Autodesk Fusion 360 part; units mm, degrees
(part 2 of 2)
sketch "Sketch11" plane through (0, 0, 0) normal (0, -1, 0) x (1, 0, 0)
  arc A0 (-10.5, 6.5391) -> (-5.9173, 0.7089) centre (-4.5, 6.5391) ccw
  arc A1 (-5.9173, 0.7089) -> (5.9173, 0.7089) centre (0, 25.0499) ccw
  arc A2 (5.9173, 0.7089) -> (10.5, 6.5391) centre (4.5, 6.5391) ccw
  line L0 (10.5, 6.5391) -> (10.5, 12.3068)
  line L1 (10.5, 12.3068) -> (-10.5, 12.3068)
  line L2 (-10.5, 12.3068) -> (-10.5, 6.5391)
  line L3 (10.5, 12.3068) -> (11.8, 12.3068)
  line L4 (13, 11.1068) -> (13, 10.9591)
  line L5 (13, 9.8068) -> (10.5, 9.8068)
  line L6 (10.5, 9.8068) -> (10.5, 12.3068)
  line L7 (12.4957, 8.7708) -> (10.4161, 4.4986)
  line L8 (0, 0) -> (3.223, 0)
  arc A3 (13, 11.1068) -> (11.8, 12.3068) centre (11.8, 11.1068) ccw
  arc A4 (12.4957, 8.7708) -> (13, 10.9591) centre (8, 10.9591) ccw
  arc A5 (3.223, 0) -> (10.4161, 4.4986) centre (3.223, 8) ccw
  circle A6 centre (11.8, 11.1068) radius 0.875
  circle A7 centre (-11.8, 11.1068) radius 0.875
  arc A8 (-13, 10.9591) -> (-12.4957, 8.7708) centre (-8, 10.9591) ccw
  line L9 (-10.5, 12.3068) -> (-11.8, 12.3068)
  arc A9 (-11.8, 12.3068) -> (-13, 11.1068) centre (-11.8, 11.1068) ccw
  line L10 (-12.4957, 8.7708) -> (-10.4161, 4.4986)
  line L11 (-13, 11.1068) -> (-13, 10.9591)
  line L12 (-13, 9.8068) -> (-10.5, 9.8068)
  arc A10 (-10.4161, 4.4986) -> (-3.223, 0) centre (-3.223, 8) ccw
  line L13 (-3.223, 0) -> (0, 0)
  line L14 (0, 0) -> (3.223, 0)
  arc A11 (3.223, 0) -> (10.4161, 4.4986) centre (3.223, 8) ccw
  line L15 (12.4957, 8.7708) -> (10.4161, 4.4986)
  arc A12 (13, 11.1068) -> (11.8, 12.3068) centre (11.8, 11.1068) ccw
  line L16 (10.5, 12.3068) -> (11.8, 12.3068)
  circle A13 centre (11.8, 11.1068) radius 0.875
  line L17 (13, 11.1068) -> (13, 10.9591)
  arc A14 (12.4957, 8.7708) -> (13, 10.9591) centre (8, 10.9591) ccw
  line L18 (10.4161, 4.4986) -> (10.907, 7.4657)
  line L19 (10.5, 9.8068) -> (10.4144, 9.8073)
  line L20 (0, 0) -> (0, 14)
  line L21 (10.2599, 10.1289) -> (10.5, 9.8068)
  arc A15 (10.907, 7.4657) -> (10.2599, 10.1289) centre (7.4539, 8.0369) ccw
  arc A16 (-10.2599, 10.1289) -> (-10.907, 7.4657) centre (-7.4539, 8.0369) ccw
  line L22 (-10.4161, 4.4986) -> (-10.907, 7.4657)
  point P0 (13, 12.3068)
  point P1 (-13, 12.3068)
  dimension "d50" = 2.5
  dimension "d51" = 2.5
  dimension "d52" = 1.2
  dimension "d53" = 5
  dimension "d54" = 8
  dimension "d55" = 1.75
  dimension "d56" = 64.044
  dimension "d60" = 115.956
  dimension "d67" = 1.2
  dimension "d68" = 5
  dimension "d69" = 8
  dimension "d70" = 1.75
  dimension "d71" = 115.956
  dimension "d73" = 16.562
  dimension "d76" = 9.5014
  dimension "d93" = 3.5
  constraint horizontal L3
  constraint vertical L4
  constraint horizontal L5
  constraint vertical L6
  constraint coincident L0.end L1.start
  constraint coincident L8.start L13.end
  constraint coincident P0 L3
  constraint coincident P0 L4
  constraint tangent L3 A3
  constraint tangent L4 A3
  constraint coincident L5.start L4
  constraint coincident L5.start L7
  constraint tangent L4 A4
  constraint tangent L7 A4
  constraint tangent L8 A5
  constraint tangent L7 A5
  constraint concentric A3 A6
  constraint tangent A1 L13
  constraint vertical A0.start L12.end
  constraint tangent A8 L11
  constraint tangent A8 L10
  constraint tangent A9 L11
  constraint tangent L9 A9
  constraint concentric A7 A9
  constraint vertical L12.start A8.start
  constraint vertical L12.start A9.end
  constraint equal A4 A8
  constraint equal A3 A9
  constraint equal L5 L12
  constraint vertical L12.start P1
  constraint tangent L10 A10
  constraint tangent A10 L13
  constraint tangent A1 L8
  constraint equal A5 A10
  constraint equal L4 L11
  constraint perpendicular L2 L9
  constraint equal L3 L9
  constraint equal A6 A7
  constraint horizontal L1.end P1
  constraint collinear L3 L9
  constraint equal L8 L13
  constraint equal L7 L10
  constraint horizontal L16
  constraint vertical L17
  constraint tangent A12 L16
  constraint tangent A12 L17
  constraint tangent L17 A14
  constraint tangent L15 A14
  constraint tangent L14 A11
  constraint tangent A11 L15
  constraint concentric A12 A13
  constraint tangent L8 A11
  constraint tangent L7 A11
  constraint tangent L3 A12
  constraint tangent L7 A14
  constraint tangent L4 A14
  constraint perpendicular L1 L20
  constraint symmetric L7.end L20 L10.end
  constraint tangent L21 A15
  constraint tangent L18 A15
  constraint symmetric L20 L21.start A16.start
  constraint symmetric L20 L18.end A16.end
  constraint symmetric L20 A15 A16
  measures "d50" distance of L0.end P0
  measures "d51" distance of L0.end L5.end
  measures "d52" radius of A3
  measures "d53" radius of A4
  measures "d54" radius of A5
  measures "d55" diameter of A6
  measures "d56" angle of L10 L12
  measures "d60" angle of L7 L8
  measures "d67" radius of A12
  measures "d68" radius of A14
  measures "d69" radius of A11
  measures "d70" diameter of A13
  measures "d71" angle of L14 L15
  measures "d73" angle of L7 L18
  measures "d76" vertical distance of L10.end L20.end
  measures "d93" radius of A15
extrude "Extrude13" add sketch "Sketch11" against normal blind 170 contours A1 A2 L0 L8 A5 L14 A11 L18 A15 | L0 L5 L7 A4 L15 A14 L18 A15 | L0 L3 L4 L5 L6 A3 A4 A12 L16 L17 A14 | A6 A13 bodies 1
extrude "Extrude14" cut sketch "Sketch11" against normal blind 110 contours L0 L5 L7 A4 L15 A14 L18 A15 | L0 L3 L4 L5 L6 A3 A4 A12 L16 L17 A14 bodies 1
extrude "Extrude15" add sketch "Sketch11" against normal blind 60 contours A1 A2 L0 L8 A5 L14 A11 L18 A15 | L0 L5 L7 A4 L15 A14 L18 A15 | L0 L3 L4 L5 L6 A3 A4 A12 L16 L17 A14 bodies 1
delete_face "DeleteFace1" 1 faces at (12.6707, 76.6667, 11.0197) on bodies 1
extrude "Extrude16" cut sketch "Sketch11" against normal blind 170 contours A6 A13 bodies 1
extrude "Extrude21" add sketch "Sketch11" against normal blind 170 contours A0 A1 L2 A10 L13 A16 L22 bodies 1
extrude "Extrude22" add sketch "Sketch11" against normal blind 110 contours L2 A8 L10 L12 A16 L22 | L2 A8 L9 A9 L11 L12 bodies 1
extrude "Extrude23" cut sketch "Sketch11" against normal blind 60 contours L2 A8 L10 L12 A16 L22 | L2 A8 L9 A9 L11 L12 bodies 1
extrude "Extrude24" add sketch "Sketch11" against normal blind 3 contours A6 A13 bodies 1
